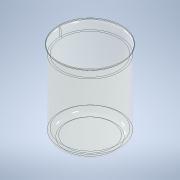
# Autodesk Inventor part: Precipitated Glass 600ml-De90-Di84-H120
Saved by Autodesk Inventor 2020 (Build 240168000, 168)
## iProperties
Created: 2020-06-20
Part Number: Precipitated Glass 600ml-De90-Di84-H120
Material: Glass
Document SubType Name: Modeling
Designer: Juan
Density: 2.18 g/cm^3
Appearance: Clear
Author: Juan
Autodesk Inventor part; units mm, degrees
ref_plane "YZ Plane" through (0, 0, 0) normal (1, 0, 0) x (0, 1, 0)
ref_plane "XZ Plane" through (0, 0, 0) normal (0, 1, 0) x (-1, 0, 0)
ref_plane "XY Plane" through (0, 0, 0) normal (0, 0, 1) x (1, 0, 0)
sketch "Sketch1" plane through (0, 0, 0) normal (0, 0, 1) x (1, 0, 0)
  line L0 (0, 0) -> (-36, 0)
  line L1 (0, 0) -> (0, 2)
  line L2 (0, 2) -> (-33, 2)
  line L3 (-45, 9) -> (-45, 118)
  line L4 (-45, 0) -> (64, 0) construction
  line L5 (-45, 118) -> (-46.5, 118)
  line L6 (-47, 118.5) -> (-47, 119.5)
  line L7 (-42, 11) -> (-42, 120)
  line L8 (-42, 120) -> (-46.5, 120)
  arc A0 (-47, 118.5) -> (-46.5, 118) centre (-46.5, 118.5) ccw
  arc A1 (-46.5, 120) -> (-47, 119.5) centre (-46.5, 119.5) ccw
  arc A2 (-42, 11) -> (-33, 2) centre (-33, 11) ccw
  arc A3 (-45, 9) -> (-36, 0) centre (-36, 9) ccw
  line L9 (-46.5, 118) -> (-45.2177, 117.872) construction
  line L10 (-45.2177, 117.872) -> (-45, 106) construction
  spline S0 degree 2 poles (-46.5, 118) (-45.2177, 117.872) (-45, 106) knots 1 1 1 2 2 2
  line L11 (-46.5, 120) -> (-42, 120) construction
  line L12 (-42, 120) -> (-42, 106) construction
  spline S1 degree 2 poles (-46.5, 120) (-42, 120) (-42, 106) knots 1 1 1 2 2 2
  point P0 (-42, 2)
  point P1 (-47, 118)
  point P2 (-47, 120)
  point P3 (-42, 106.0002)
  dimension "d0" = 45
  dimension "d1" = 2
  dimension "d2" = 42
  dimension "d3" = 90
  dimension "d4" = 118
  dimension "d5" = 90
  dimension "d6" = 2
  dimension "d7" = 2
  dimension "d8" = 90
  dimension "d9" = 12
  dimension "d10" = 0.5
  dimension "d11" = 0.5
  dimension "d12" = 9
  dimension "d13" = 9
  constraints: 18 end point, 10 point on line, 8 point on circle, 8 tangent, 5 perpendicular, 4 centre point, 3 vertical, 2 horizontal, 1 coincident, 6 other
  measures "d0" distance of L0.start L4.start
  measures "d1" distance of L0.start L1.end
  measures "d2" distance of L1.end point (-42, 2)
  measures "d3" angle of L2 L1
  measures "d4" distance of L4.start L3.end
  measures "d5" angle of L4 L3
  measures "d6" distance of L3.end point (-47, 118)
  measures "d7" distance of point (-47, 118) point (-47, 120)
  measures "d8" angle of L5 L6
  measures "d9" distance from line of L5 L10.end
  measures "d10" radius of A0
  measures "d11" radius of A1
  measures "d12" radius of A2
  measures "d13" radius of A3
revolve "Revolution1" add sketch "Sketch1" angle 360 about axis through (0, 0, 0) along (0, 1, 0) contours L0 A3 L3 L5 A0 L6 A1 S1 L7 A2 L2 L1 | S0 L5 L3
body "Solid1"
